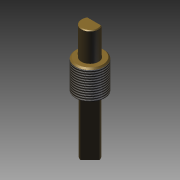
# Autodesk Inventor part: HS13Z-D-shaft
Saved by Autodesk Inventor 2011 SP1 (Build 150282100, 282)
## iProperties
Created: 2016-09-01
Part Number: HS13Z-D-shaft
Catalog Web Link: www.cadenas.de
Description: HS Series - 6 AMP Single Pole Standard Size Rotaries -shaft-
Vendor: NKKSWITCHES
Document SubType Name: Modeling
Designer: psAdmin
Manufacturer: NKKSWITCHES
Mass: 1.32957 g
Surface Area: 9.62054 cm^2
Volume: 1.32957 cm^3
Density: 1 g/cm^3
Category: PARTsolutions
Company: NKKSWITCHES
Title: HS13Z-D-shaft
Author: Cadenas PARTsolutions
PSOL_IDENT_0: {$CADENAS_DATA\23d-libs\nkkswitches\rotary\hs_12_amp\parts\hs_6amp_shaft.prj},226 {VTYP=3D},{NB=HS13
PSOL_IDENT_1: Z-D-shaft},{LINA=HS13Z-D-shaft},{NN=HS Series - 6 AMP Single Pole Standard Size Rotaries -shaft},{DA
PSOL_IDENT_2: TE=22.09.2015 06:04:15},{GEOMDATE=09.04.2009 06:16:00},{VERSION=},{LINEID=30},{LINESUBID=-1},{WBVAR=
PSOL_IDENT_3: SHAFT}  {NB=HS13Z-D-shaft},{LINA=HS13Z-D-shaft},{KT=DUMMY},{PN=HS13Z-D},{SRS=HS},{MDL=HS13Z},{SHAFT=
PSOL_IDENT_4: -D},{ND=10},{PITCH=0.75}
NN: HS Series - 6 AMP Single Pole Standard Size Rotaries -shaft
NB: HS13Z-D-shaft
NBSYN: $PN.-shaft
LINA: HS13Z-D-shaft
PN: HS13Z-D
SRS: HS
MDL: HS13Z
SHAFT: D - D-flat Shaft
ND: 10
PITCH: 0.75
SUPPLIER: NKKSWITCHES
ARTICLENO: HS13Z-D-shaft
BOMINFO: HS13Z-D-shaft
CREATOR: CADENAS GmbH
Autodesk Inventor part; units mm, degrees
sketch "Sketch_2" plane through (0, 0, 0) normal (1, 0, 0) x (0, 1, 0)
  line L0 (0, 0) -> (20.0152, 0)
  line L1 (20.0152, 0) -> (20.0152, -2.7432)
  line L2 (20.0152, -2.7432) -> (19.7612, -2.9972)
  line L3 (19.7612, -2.9972) -> (10.0076, -2.9972)
  line L4 (10.0076, -2.9972) -> (10.0076, -4.54)
  line L5 (10.0076, -4.54) -> (9.5476, -5)
  line L6 (9.5476, -5) -> (0, -5)
  line L7 (0, -5) -> (0, 0)
  line L8 (0, 0) -> (20.0152, 0)
  constraints: 18 end point
revolve "Revolution1" add sketch "Sketch_2" angle 360 about axis through (0, 0, 0) along (0, -1, 0)
thread "Thread1" size "M10x0.75" class "6g" standard "ISO Metric profile" full length
sketch "Sketch_3" plane through (0, 20.0152, 0) normal (0, 1, 0) x (1, 0, 0)
  line L0 (-2.6517, 1.397) -> (2.6517, 1.397)
  arc A0 (2.6517, 1.397) -> (-2.6517, 1.397) centre (0, 0) ccw
  constraints: 2 end point, 2 point on circle, 1 centre point
extrude "Extrusion1" cut sketch "Sketch_3" against normal blind 9.0678
sketch "Sketch_5" plane through (0, 0, 0) normal (0, 1, 0) x (-1, 0, 0)
  arc A0 (2.7335, 0.5782) -> (0.5782, 2.7335) centre (0, 0) ccw
  line L0 (0.5782, 2.7335) -> (-2.7335, -0.5782)
  arc A1 (-2.7335, -0.5782) -> (-0.5782, -2.7335) centre (0, 0) ccw
  line L1 (-0.5782, -2.7335) -> (2.7335, 0.5782)
  constraints: 4 end point, 4 point on circle, 2 centre point
extrude "Extrusion2" add sketch "Sketch_5" against normal blind 19.9898
sketch "Sketch_10" plane through (0, 0, 0) normal (0, 1, 0) x (-1, 0, 0)
  line L0 (4.0411, -3.5023) -> (3.5023, -2.9635)
  line L1 (3.5023, -2.9635) -> (2.9635, -3.5023)
  line L2 (2.9635, -3.5023) -> (3.5023, -4.0411)
  line L3 (3.5023, -4.0411) -> (4.0411, -3.5023)
  constraints: 8 end point
extrude "Extrusion3" cut sketch "Sketch_10" along normal blind 25.4
ref_plane "at518_XY" through (0, 3.4925, 0) normal (0, -1, 0) x (1, 0, 0)
ref_plane "at518_YZ" through (0, 3.4925, 0) normal (1, 0, 0) x (0, 0, 1)
ref_plane "at518_ZX" through (0, 3.4925, 0) normal (0, 0, 1) x (0, -1, 0)
ref_plane "at520_XY" through (0, 2.5019, 0) normal (0, -1, 0) x (1, 0, 0)
ref_plane "at520_YZ" through (0, 2.5019, 0) normal (1, 0, 0) x (0, 0, 1)
ref_plane "at520_ZX" through (0, 2.5019, 0) normal (0, 0, 1) x (0, -1, 0)
ref_plane "at526_a_XY" through (0, 1.0033, 0) normal (0, -1, 0) x (1, 0, 0)
ref_plane "at526_a_YZ" through (0, 1.0033, 0) normal (1, 0, 0) x (0, 0, 1)
ref_plane "at526_a_ZX" through (0, 1.0033, 0) normal (0, 0, 1) x (0, -1, 0)
ref_plane "at526_b_XY" through (0, 4.9911, 0) normal (0, -1, 0) x (1, 0, 0)
ref_plane "at526_b_YZ" through (0, 4.9911, 0) normal (1, 0, 0) x (0, 0, 1)
ref_plane "at526_b_ZX" through (0, 4.9911, 0) normal (0, 0, 1) x (0, -1, 0)
ref_plane "to_body_XY" through (0, 0, 0) normal (0, 1, 0) x (1, 0, 0)
ref_plane "to_body_YZ" through (0, 0, 0) normal (1, 0, 0) x (0, 0, -1)
ref_plane "to_body_ZX" through (0, 0, 0) normal (0, 0, -1) x (0, 1, 0)
body "Solid1"
